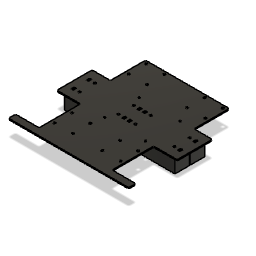
pcb v49 (Autodesk Fusion 360 design; units mm, degrees)
Autodesk Fusion 360 part; units mm, degrees
sketch "Sketch4" plane through (0, 0, 0) normal (0, 1, 0) x (1, 0, 0)
  line L0 (0, 0) -> (0, -168.9)
  circle A0 centre (28.5, -28.9) radius 1.6
  circle A1 centre (54.5, -4) radius 1.6
  circle A2 centre (21, -117) radius 1.6
  circle A3 centre (47, -141.9) radius 1.6
  line L1 (85.5, -50) -> (85.5, -100)
  line L2 (52, -158.9) -> (85.5, -158.9)
  line L3 (52, -100) -> (52, -158.9)
  circle A4 centre (47, -117) radius 1.6
  circle A5 centre (28.5, -4) radius 1.6
  line L4 (59.5, -50) -> (85.5, -50)
  circle A6 centre (54.5, -28.9) radius 1.6
  line L5 (59.5, 0) -> (59.5, -50)
  line L6 (85.5, -158.9) -> (85.5, -168.9)
  circle A7 centre (21, -141.9) radius 1.6
  line L7 (85.5, -168.9) -> (0, -168.9)
  line L8 (0, 0) -> (59.5, 0)
  line L9 (85.5, -100) -> (52, -100)
  line L10 (0, 0) -> (-59.5, 0)
  line L11 (-59.5, 0) -> (-59.5, -50)
  line L12 (-59.5, -50) -> (-85.5, -50)
  line L13 (-85.5, -50) -> (-85.5, -100)
  line L14 (-85.5, -100) -> (-52, -100)
  line L15 (-52, -100) -> (-52, -158.9)
  line L16 (-52, -158.9) -> (-85.5, -158.9)
  line L17 (-85.5, -158.9) -> (-85.5, -168.9)
  line L18 (-85.5, -168.9) -> (0, -168.9)
  line L19 (-85.5, -75) -> (85.5, -75) construction
  circle A8 centre (-28.5, -28.9) radius 1.6
  circle A9 centre (-28.5, -4) radius 1.6
  circle A10 centre (-54.5, -28.9) radius 1.6
  circle A11 centre (-54.5, -4) radius 1.6
  circle A12 centre (-21, -117) radius 1.6
  circle A13 centre (-47, -117) radius 1.6
  circle A14 centre (-47, -141.9) radius 1.6
  circle A15 centre (-21, -141.9) radius 1.6
  circle A16 centre (57.5, -2) radius 2
  circle A17 centre (61, -48.5) radius 1.5
  circle A18 centre (83.5, -52) radius 2
  circle A19 centre (83.5, -98) radius 2
  circle A20 centre (53.5, -101.5) radius 1.5
  circle A21 centre (53.5, -157.4) radius 1.5
  circle A22 centre (83.5, -160.9) radius 2
  circle A23 centre (83.5, -166.9) radius 2
  circle A24 centre (-57.5, -2) radius 2
  circle A25 centre (-61, -48.5) radius 1.5
  circle A26 centre (-83.5, -52) radius 2
  circle A27 centre (-83.5, -98) radius 2
  circle A28 centre (-53.5, -101.5) radius 1.5
  circle A29 centre (-53.5, -157.4) radius 1.5
  circle A30 centre (-83.5, -160.9) radius 2
  circle A31 centre (-83.5, -166.9) radius 2
  circle A32 centre (-18, -50.5) radius 1.4
  circle A33 centre (40, -50.5) radius 1.4
  circle A34 centre (40, -99.5) radius 1.4
  circle A35 centre (-18, -99.5) radius 1.4
  line L20 (-41.5, -103) -> (-41.5, -47)
  line L21 (43.5, -103) -> (-41.5, -103)
  line L22 (43.5, -47) -> (43.5, -103)
  line L23 (-41.5, -47) -> (43.5, -47)
  line L24 (1, -53.8) -> (78.47, -53.8)
  line L25 (78.47, -53.8) -> (78.47, -74.5)
  line L26 (78.47, -74.5) -> (1, -74.5)
  line L27 (1, -74.5) -> (1, -53.8)
  circle A36 centre (12.11, -64.15) radius 1.6
  circle A37 centre (67.36, -64.15) radius 1.6
  line L28 (2.335, -62.05) -> (5.335, -62.05)
  line L29 (5.335, -62.05) -> (5.335, -66.25)
  line L30 (5.335, -66.25) -> (2.335, -66.25)
  line L31 (2.335, -66.25) -> (2.335, -62.05)
  line L32 (74.135, -62.05) -> (77.135, -62.05)
  line L33 (77.135, -62.05) -> (77.135, -66.25)
  line L34 (77.135, -66.25) -> (74.135, -66.25)
  line L35 (74.135, -66.25) -> (74.135, -62.05)
  line L36 (74.135, -83.75) -> (77.135, -83.75)
  line L37 (2.335, -83.75) -> (5.335, -83.75)
  circle A38 centre (67.36, -85.85) radius 1.6
  line L38 (77.135, -87.95) -> (74.135, -87.95)
  line L39 (5.335, -83.75) -> (5.335, -87.95)
  line L40 (5.335, -87.95) -> (2.335, -87.95)
  line L41 (77.135, -83.75) -> (77.135, -87.95)
  line L42 (74.135, -87.95) -> (74.135, -83.75)
  line L43 (1, -75.5) -> (78.47, -75.5)
  line L44 (1, -96.2) -> (1, -75.5)
  circle A39 centre (12.11, -85.85) radius 1.6
  line L45 (78.47, -75.5) -> (78.47, -96.2)
  line L46 (2.335, -87.95) -> (2.335, -83.75)
  line L47 (78.47, -96.2) -> (1, -96.2)
  line L48 (-74.135, -62.05) -> (-74.135, -66.25)
  circle A40 centre (-67.36, -64.15) radius 1.6
  line L49 (-5.335, -83.75) -> (-2.335, -83.75)
  line L50 (-1, -96.2) -> (-78.47, -96.2)
  line L51 (-5.335, -66.25) -> (-5.335, -62.05)
  circle A41 centre (-67.36, -85.85) radius 1.6
  line L52 (-77.135, -62.05) -> (-74.135, -62.05)
  line L53 (-77.135, -66.25) -> (-77.135, -62.05)
  line L54 (-74.135, -66.25) -> (-77.135, -66.25)
  line L55 (-2.335, -83.75) -> (-2.335, -87.95)
  circle A42 centre (-12.11, -64.15) radius 1.6
  line L56 (-78.47, -53.8) -> (-1, -53.8)
  line L57 (-74.135, -83.75) -> (-74.135, -87.95)
  line L58 (-78.47, -74.5) -> (-78.47, -53.8)
  line L59 (-1, -53.8) -> (-1, -74.5)
  line L60 (-2.335, -62.05) -> (-2.335, -66.25)
  line L61 (-77.135, -83.75) -> (-74.135, -83.75)
  line L62 (-2.335, -66.25) -> (-5.335, -66.25)
  line L63 (-74.135, -87.95) -> (-77.135, -87.95)
  line L64 (-78.47, -75.5) -> (-1, -75.5)
  line L65 (-5.335, -87.95) -> (-5.335, -83.75)
  line L66 (-77.135, -87.95) -> (-77.135, -83.75)
  circle A43 centre (-12.11, -85.85) radius 1.6
  line L67 (-5.335, -62.05) -> (-2.335, -62.05)
  line L68 (-1, -74.5) -> (-78.47, -74.5)
  line L69 (-2.335, -87.95) -> (-5.335, -87.95)
  line L70 (-78.47, -96.2) -> (-78.47, -75.5)
  line L71 (-1, -75.5) -> (-1, -96.2)
  line L72 (-39.735, -53.8) -> (-39.735, -96.2) construction
  point P0 (0, -168.9)
  dimension "d52" = 50
  dimension "d53" = 26
  dimension "d54" = 50
  dimension "d55" = 33.5
  dimension "d56" = 58.9
  dimension "d57" = 3.2
  dimension "d58" = 3.2
  dimension "d59" = 3.2
  dimension "d60" = 3.2
  dimension "d61" = 24.9
  dimension "d62" = 24.9
  dimension "d63" = 26
  dimension "d64" = 26
  dimension "d65" = 17
  dimension "d66" = 17
  dimension "d67" = 5
  dimension "d68" = 5
  dimension "d69" = 33.5
  dimension "d70" = 10
  dimension "d71" = 3.2
  dimension "d72" = 3.2
  dimension "d73" = 3.2
  dimension "d74" = 3.2
  dimension "d75" = 24.9
  dimension "d76" = 24.9
  dimension "d77" = 26
  dimension "d78" = 26
  dimension "d79" = 59.5
  dimension "d80" = 85.5
  dimension "d81" = 4
  dimension "d82" = 5
  dimension "d83" = 5
  dimension "d84" = 4
  dimension "d165" = 4
  dimension "d166" = 2
  dimension "d167" = 2
  dimension "d168" = 3
  dimension "d171" = 1.5
  dimension "d172" = 1.5
  dimension "d173" = 4
  dimension "d174" = 2
  dimension "d175" = 2
  dimension "d176" = 4
  dimension "d177" = 2
  dimension "d178" = 2
  dimension "d179" = 3
  dimension "d180" = 1.5
  dimension "d181" = 1.5
  dimension "d182" = 3
  dimension "d183" = 1.5
  dimension "d184" = 1.5
  dimension "d185" = 4
  dimension "d186" = 2
  dimension "d187" = 2
  dimension "d188" = 4
  dimension "d189" = 2
  dimension "d190" = 2
  dimension "d191" = 85
  dimension "d192" = 56
  dimension "d193" = 2.8
  dimension "d194" = 3.5
  dimension "d195" = 3.5
  dimension "d196" = 2.8
  dimension "d197" = 3.5
  dimension "d198" = 2.8
  dimension "d199" = 2.8
  dimension "d200" = 3.5
  dimension "d201" = 58
  dimension "d202" = 58
  dimension "d203" = 49
  dimension "d204" = 49
  dimension "d205" = 12
  dimension "d206" = 77.47
  dimension "d207" = 20.7
  dimension "d208" = 3.2
  dimension "d209" = 3.2
  dimension "d210" = 55.25
  dimension "d211" = 10.35
  dimension "d212" = 10.35
  dimension "d213" = 11.11
  dimension "d214" = 3
  dimension "d215" = 4.2
  dimension "d216" = 3
  dimension "d217" = 4.2
  dimension "d218" = 8.25
  dimension "d219" = 1.335
  dimension "d220" = 8.25
  dimension "d221" = 1.335
  dimension "d222" = 77.47
  dimension "d223" = 20.7
  dimension "d224" = 3.2
  dimension "d225" = 3.2
  dimension "d226" = 55.25
  dimension "d227" = 10.35
  dimension "d228" = 10.35
  dimension "d229" = 11.11
  dimension "d230" = 3
  dimension "d231" = 4.2
  dimension "d232" = 3
  dimension "d233" = 4.2
  dimension "d234" = 8.25
  dimension "d235" = 1.335
  dimension "d236" = 8.25
  dimension "d237" = 1.335
  dimension "d238" = 1
  dimension "d239" = 0
  dimension "d240" = 77.47
  dimension "d241" = 20.7
  dimension "d242" = 3.2
  dimension "d243" = 3.2
  dimension "d244" = 55.25
  dimension "d245" = 10.35
  dimension "d246" = 10.35
  dimension "d247" = 11.11
  dimension "d248" = 3
  dimension "d249" = 4.2
  dimension "d250" = 3
  dimension "d251" = 4.2
  dimension "d252" = 8.25
  dimension "d253" = 1.335
  dimension "d254" = 8.25
  dimension "d255" = 1.335
  dimension "d256" = 77.47
  dimension "d257" = 20.7
  dimension "d258" = 3.2
  dimension "d259" = 3.2
  dimension "d260" = 55.25
  dimension "d261" = 10.35
  dimension "d262" = 10.35
  dimension "d263" = 11.11
  dimension "d264" = 3
  dimension "d265" = 4.2
  dimension "d266" = 3
  dimension "d267" = 4.2
  dimension "d268" = 8.25
  dimension "d269" = 1.335
  dimension "d270" = 8.25
  dimension "d271" = 1.335
  dimension "d272" = 1
  dimension "d273" = 0
  dimension "d274" = 2
  constraint horizontal L8
  constraint perpendicular L5 L8
  constraint perpendicular L4 L5
  constraint vertical L1
  constraint perpendicular L1 L9
  constraint perpendicular L3 L9
  constraint perpendicular L2 L3
  constraint perpendicular L2 L6
  constraint perpendicular L6 L7
  constraint coincident P0 L0.end
  constraint coincident L0.start L8.start
  constraint symmetric L8.start L0 L10.start
  constraint symmetric L5.start L0 L10.end
  constraint symmetric L4.start L0 L11.end
  constraint symmetric L1.start L0 L12.end
  constraint symmetric L1.end L0 L13.end
  constraint symmetric L3.start L0 L14.end
  constraint symmetric L2.start L0 L15.end
  constraint symmetric L2.end L0 L16.end
  constraint symmetric L6.end L0 L17.end
  constraint symmetric P0 L0 L7.end
  constraint midpoint L13 L19.start
  constraint midpoint L1 L19.end
  constraint symmetric L0 A0 A8
  constraint symmetric L0 A1 A11
  constraint symmetric L0 A2 A12
  constraint symmetric L0 A3 A14
  constraint symmetric L0 A4 A13
  constraint symmetric L0 A5 A9
  constraint symmetric L0 A6 A10
  constraint symmetric L0 A7 A15
  constraint symmetric L0 A16 A24
  constraint symmetric L0 A17 A25
  constraint symmetric L0 A18 A26
  constraint symmetric L0 A19 A27
  constraint symmetric L0 A20 A28
  constraint symmetric L0 A21 A29
  constraint symmetric L0 A22 A30
  constraint symmetric L0 A23 A31
  constraint vertical L22
  constraint horizontal L23
  constraint horizontal L21
  constraint perpendicular L20 L23
  constraint symmetric L19 L21 L23
  constraint horizontal L24
  constraint vertical L25
  constraint horizontal L26
  constraint vertical L27
  constraint horizontal L28
  constraint vertical L29
  constraint horizontal L30
  constraint vertical L31
  constraint horizontal L32
  constraint vertical L33
  constraint horizontal L34
  constraint vertical L35
  constraint horizontal L43
  constraint vertical L45
  constraint horizontal L47
  constraint vertical L44
  constraint horizontal L37
  constraint vertical L39
  constraint horizontal L40
  constraint vertical L46
  constraint horizontal L36
  constraint vertical L41
  constraint horizontal L38
  constraint vertical L42
  constraint horizontal L56
  constraint vertical L59
  constraint horizontal L68
  constraint vertical L58
  constraint horizontal L52
  constraint vertical L48
  constraint horizontal L54
  constraint vertical L53
  constraint horizontal L67
  constraint vertical L60
  constraint horizontal L62
  constraint vertical L51
  constraint horizontal L64
  constraint vertical L71
  constraint horizontal L50
  constraint vertical L70
  constraint horizontal L61
  constraint vertical L57
  constraint horizontal L63
  constraint vertical L66
  constraint horizontal L49
  constraint vertical L55
  constraint horizontal L69
  constraint vertical L65
  constraint collinear L24 L56
  constraint symmetric L19 L50 L56
  constraint midpoint L56 L72.start
  constraint midpoint L50 L72.end
  measures "d52" distance of L5.start L4.start
  measures "d53" distance of L4.start L1.start
  measures "d54" distance of L1.start L1.end
  measures "d55" distance of L1.end L3.start
  measures "d56" distance of L3.start L2.start
  measures "d57" diameter of A4
  measures "d58" diameter of A2
  measures "d59" diameter of A3
  measures "d60" diameter of A7
  measures "d61" vertical distance of A4.centre A3.centre
  measures "d62" vertical distance of A2.centre A7.centre
  measures "d63" horizontal distance of A4.centre A2.centre
  measures "d64" horizontal distance of A3.centre A7.centre
  measures "d65" vertical distance of A4.centre L3.start
  measures "d66" vertical distance of L3.start A2.centre
  measures "d67" distance of A3.centre L3
  measures "d68" distance of A4.centre L3
  measures "d69" distance of L2.start L2.end
  measures "d70" distance of L2.end L6.end
  measures "d71" diameter of A1
  measures "d72" diameter of A5
  measures "d73" diameter of A6
  measures "d74" diameter of A0
  measures "d75" vertical distance of A6.centre A1.centre
  measures "d76" vertical distance of A0.centre A5.centre
  measures "d77" horizontal distance of A5.centre A1.centre
  measures "d78" horizontal distance of A0.centre A6.centre
  measures "d79" distance of L0.start L5.start
  measures "d80" distance of L6.end P0
  measures "d81" distance of A1.centre L8
  measures "d82" distance of A1.centre L5
  measures "d83" distance of A6.centre L5
  measures "d84" distance of A5.centre L8
  measures "d165" diameter of A16
  measures "d166" distance of L8 A16.centre
  measures "d167" distance of L5 A16.centre
  measures "d168" diameter of A17
  measures "d171" distance of L5 A17.centre
  measures "d172" distance of L4 A17.centre
  measures "d173" diameter of A18
  measures "d174" distance of L4 A18.centre
  measures "d175" distance of L1 A18.centre
  measures "d176" diameter of A19
  measures "d177" distance of L9 A19.centre
  measures "d178" distance of L1 A19.centre
  measures "d179" diameter of A20
  measures "d180" distance of L9 A20.centre
  measures "d181" distance of L3 A20.centre
  measures "d182" diameter of A21
  measures "d183" distance of L3 A21.centre
  measures "d184" distance of L2 A21.centre
  measures "d185" diameter of A22
  measures "d186" distance of L2 A22.centre
  measures "d187" distance of L6 A22.centre
  measures "d188" diameter of A23
  measures "d189" distance of L7 A23.centre
  measures "d190" distance of L6 A23.centre
  measures "d191" distance of L21.start L20.start
  measures "d192" distance of L21.start L22.start
  measures "d193" diameter of A34
  measures "d194" distance of A34.centre L21
  measures "d195" distance of A34.centre L22
  measures "d196" diameter of A33
  measures "d197" distance of A33.centre L22
  measures "d198" diameter of A35
  measures "d199" diameter of A32
  measures "d200" distance of A35.centre L21
  measures "d201" distance of A35.centre A34.centre
  measures "d202" distance of A32.centre A33.centre
  measures "d203" distance of A33.centre A34.centre
  measures "d204" distance of A32.centre A35.centre
  measures "d205" distance of L3 A34.centre
  measures "d206" distance of L24.start L24.end
  measures "d207" distance of L24.start L26.end
  measures "d208" diameter of A36
  measures "d209" diameter of A37
  measures "d210" horizontal distance of A36.centre A37.centre
  measures "d211" distance of L26 A36.centre
  measures "d212" distance of L26 A37.centre
  measures "d213" distance of L27 A36.centre
  measures "d214" distance of L28.start L28.end
  measures "d215" distance of L28.start L30.end
  measures "d216" distance of L32.start L32.end
  measures "d217" distance of L32.start L34.end
  measures "d218" distance of L24 L32
  measures "d219" distance of L25 L33
  measures "d220" distance of L24 L28
  measures "d221" distance of L27 L31
  measures "d222" distance of L43.start L43.end
  measures "d223" distance of L43.start L44.start
  measures "d224" diameter of A39
  measures "d225" diameter of A38
  measures "d226" horizontal distance of A39.centre A38.centre
  measures "d227" distance of A39.centre L47
  measures "d228" distance of A38.centre L47
  measures "d229" distance of A39.centre L44
  measures "d230" distance of L37.start L37.end
  measures "d231" distance of L37.start L40.end
  measures "d232" distance of L36.end L36.start
  measures "d233" distance of L38.end L36.start
  measures "d234" distance of L36 L43
  measures "d235" distance of L41 L45
  measures "d236" distance of L37 L43
  measures "d237" distance of L44 L46
  measures "d238" distance of L26 L43
  measures "d239" distance of L25 L45
  measures "d240" distance of L56.start L56.end
  measures "d241" distance of L56.start L58.start
  measures "d242" diameter of A40
  measures "d243" diameter of A42
  measures "d244" horizontal distance of A40.centre A42.centre
  measures "d245" distance of A40.centre L68
  measures "d246" distance of A42.centre L68
  measures "d247" distance of A40.centre L58
  measures "d248" distance of L52.start L48.start
  measures "d249" distance of L52.start L53.start
  measures "d250" distance of L60.start L51.end
  measures "d251" distance of L51.start L51.end
  measures "d252" distance of L56 L67
  measures "d253" distance of L59 L60
  measures "d254" distance of L52 L56
  measures "d255" distance of L53 L58
  measures "d256" distance of L64.start L64.end
  measures "d257" distance of L64.start L50.end
  measures "d258" diameter of A41
  measures "d259" diameter of A43
  measures "d260" horizontal distance of A43.centre A41.centre
  measures "d261" distance of A41.centre L50
  measures "d262" distance of A43.centre L50
  measures "d263" distance of A41.centre L70
  measures "d264" distance of L57.start L61.start
  measures "d265" distance of L61.start L63.end
  measures "d266" distance of L49.start L49.end
  measures "d267" distance of L65.start L49.start
  measures "d268" distance of L49 L64
  measures "d269" distance of L55 L71
  measures "d270" distance of L61 L64
  measures "d271" distance of L66 L70
  measures "d272" distance of L64 L68
  measures "d273" distance of L59 L71
  measures "d274" distance of L27 L59
extrude "Extrude8" add sketch "Sketch4" along normal blind 1.6 contours L0 L1 L2 L3 L4 L5 L6 L7 L8 L9 A16 A18 A19 A22 A23 L21 L22 L23 L24 L25 L26 L43 L45 L47 | L0 L10 L11 L12 L13 L14 L15 L16 L17 L18 A24 A26 A27 A30 A31 L20 L21 L23 L50 L56 L58 L64 L68 L70 | L0 L21 L22 L23 L24 L26 L27 L43 L44 L47 | L0 L20 L21 L23 L50 L56 L59 L64 L68 L71 | A16 | A24 | L20 L56 L59 L68 | L20 L56 L58 L68 | L22 L24 L25 L26 | L22 L24 L26 L27 | L4 L5 A17 | L11 L12 A25 | A23 | A31 | L22 L43 L44 L47 | L22 L43 L45 L47 | L20 L50 L64 L70 | L20 L50 L64 L71 | A18 | A26 | A22 | A30 | A19 | A27 | L2 L3 A21 | L15 L16 A29 | L3 L9 A20 | L14 L15 A28 makes body 1
extrude "Extrude11" add sketch "Sketch4" against normal blind 21.4 separate body contours L20 L56 L59 L68 | L20 L56 L58 L68 | L22 L24 L25 L26 | L22 L24 L26 L27 | L22 L43 L44 L47 | L22 L43 L45 L47 | L20 L50 L64 L70 | L20 L50 L64 L71 makes body 2 at (-26.8233, -14.2667, 75.5) makes body 3 at (52.6467, -7.1333, 96.2) makes body 4 at (-26.8233, -7.1333, 74.5) makes body 5 at (26.8233, -7.1333, 53.8)
sketch "Sketch9" plane through (0, 1.6, 0) normal (0, 1, 0) x (-1, 0, 0)
  line L0 (2.335, 83.75) -> (2.335, 87.95)
  line L1 (2.335, 87.95) -> (5.335, 87.95)
  line L2 (5.335, 87.95) -> (5.335, 83.75)
  line L3 (5.335, 83.75) -> (2.335, 83.75)
  circle A0 centre (12.11, 85.85) radius 1.6
  line L4 (5.335, 66.25) -> (5.335, 62.05)
  line L5 (5.335, 62.05) -> (2.335, 62.05)
  line L6 (2.335, 62.05) -> (2.335, 66.25)
  line L7 (2.335, 66.25) -> (5.335, 66.25)
  line L8 (74.135, 87.95) -> (77.135, 87.95)
  line L9 (77.135, 87.95) -> (77.135, 83.75)
  line L10 (77.135, 83.75) -> (74.135, 83.75)
  line L11 (74.135, 83.75) -> (74.135, 87.95)
  circle A1 centre (-67.36, 64.15) radius 1.6
  circle A2 centre (-12.11, 64.15) radius 1.6
  circle A3 centre (-40, 50.5) radius 1.4
  circle A4 centre (18, 99.5) radius 1.4
  circle A5 centre (-40, 99.5) radius 1.4
  line L12 (-5.335, 66.25) -> (-2.335, 66.25)
  line L13 (-2.335, 66.25) -> (-2.335, 62.05)
  line L14 (-2.335, 62.05) -> (-5.335, 62.05)
  line L15 (-5.335, 62.05) -> (-5.335, 66.25)
  circle A6 centre (-54.5, 28.9) radius 1.6
  circle A7 centre (-28.5, 4) radius 1.6
  circle A8 centre (-28.5, 28.9) radius 1.6
  circle A9 centre (-47, 117) radius 1.6
  circle A10 centre (-54.5, 4) radius 1.6
  circle A11 centre (-21, 117) radius 1.6
  circle A12 centre (-47, 141.9) radius 1.6
  circle A13 centre (18, 50.5) radius 1.4
  circle A14 centre (-12.11, 85.85) radius 1.6
  circle A15 centre (67.36, 85.85) radius 1.6
  circle A16 centre (67.36, 64.15) radius 1.6
  circle A17 centre (28.5, 28.9) radius 1.6
  circle A18 centre (28.5, 4) radius 1.6
  circle A19 centre (54.5, 4) radius 1.6
  circle A20 centre (21, 117) radius 1.6
  circle A21 centre (54.5, 28.9) radius 1.6
  circle A22 centre (47, 117) radius 1.6
  line L16 (-77.135, 87.95) -> (-74.135, 87.95)
  line L17 (-74.135, 87.95) -> (-74.135, 83.75)
  line L18 (-74.135, 83.75) -> (-77.135, 83.75)
  line L19 (-77.135, 83.75) -> (-77.135, 87.95)
  line L20 (-77.135, 66.25) -> (-74.135, 66.25)
  line L21 (-74.135, 66.25) -> (-74.135, 62.05)
  line L22 (-74.135, 62.05) -> (-77.135, 62.05)
  line L23 (-77.135, 62.05) -> (-77.135, 66.25)
  circle A23 centre (21, 141.9) radius 1.6
  circle A24 centre (47, 141.9) radius 1.6
  circle A25 centre (12.11, 64.15) radius 1.6
  line L24 (74.135, 62.05) -> (74.135, 66.25)
  line L25 (74.135, 66.25) -> (77.135, 66.25)
  line L26 (77.135, 66.25) -> (77.135, 62.05)
  line L27 (77.135, 62.05) -> (74.135, 62.05)
  circle A26 centre (-21, 141.9) radius 1.6
  line L28 (-5.335, 87.95) -> (-2.335, 87.95)
  line L29 (-2.335, 87.95) -> (-2.335, 83.75)
  line L30 (-2.335, 83.75) -> (-5.335, 83.75)
  line L31 (-5.335, 83.75) -> (-5.335, 87.95)
  circle A27 centre (-67.36, 85.85) radius 1.6
  line L32 (53.5, 158.9) -> (83.5, 158.9)
  arc A28 (83.5, 158.9) -> (85.5, 160.9) centre (83.5, 160.9) ccw
  line L33 (85.5, 160.9) -> (85.5, 166.9)
  arc A29 (85.5, 166.9) -> (83.5, 168.9) centre (83.5, 166.9) ccw
  line L34 (83.5, 168.9) -> (-83.5, 168.9)
  arc A30 (-83.5, 168.9) -> (-85.5, 166.9) centre (-83.5, 166.9) ccw
  line L35 (-85.5, 166.9) -> (-85.5, 160.9)
  arc A31 (-85.5, 160.9) -> (-83.5, 158.9) centre (-83.5, 160.9) ccw
  line L36 (-83.5, 158.9) -> (-53.5, 158.9)
  arc A32 (-52, 157.4) -> (-53.5, 158.9) centre (-53.5, 157.4) ccw
  line L37 (-52, 157.4) -> (-52, 101.5)
  arc A33 (-53.5, 100) -> (-52, 101.5) centre (-53.5, 101.5) ccw
  line L38 (-53.5, 100) -> (-83.5, 100)
  arc A34 (-83.5, 100) -> (-85.5, 98) centre (-83.5, 98) ccw
  line L39 (-85.5, 98) -> (-85.5, 52)
  arc A35 (-85.5, 52) -> (-83.5, 50) centre (-83.5, 52) ccw
  line L40 (-83.5, 50) -> (-61, 50)
  arc A36 (-59.5, 48.5) -> (-61, 50) centre (-61, 48.5) ccw
  line L41 (-59.5, 48.5) -> (-59.5, 2)
  arc A37 (-59.5, 2) -> (-57.5, 0) centre (-57.5, 2) ccw
  line L42 (-57.5, 0) -> (57.5, 0)
  arc A38 (57.5, 0) -> (59.5, 2) centre (57.5, 2) ccw
  line L43 (59.5, 2) -> (59.5, 48.5)
  arc A39 (61, 50) -> (59.5, 48.5) centre (61, 48.5) ccw
  line L44 (61, 50) -> (83.5, 50)
  arc A40 (83.5, 50) -> (85.5, 52) centre (83.5, 52) ccw
  line L45 (85.5, 52) -> (85.5, 98)
  arc A41 (85.5, 98) -> (83.5, 100) centre (83.5, 98) ccw
  line L46 (83.5, 100) -> (53.5, 100)
  arc A42 (52, 101.5) -> (53.5, 100) centre (53.5, 101.5) ccw
  line L47 (52, 101.5) -> (52, 157.4)
  arc A43 (53.5, 158.9) -> (52, 157.4) centre (53.5, 157.4) ccw
